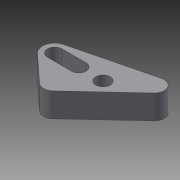
# Autodesk Inventor part: brake
Saved by Autodesk Inventor 2018 (Build 220112000, 112)
## iProperties
Created: 2019-02-20
Part Number: brake
Material: 一般
Document SubType Name: Modeling
Designer: ku_sk
Density: 1 g/cm^3
Appearance: 既定
Author: ku_sk
Autodesk Inventor part; units mm, degrees
ref_plane "YZ Plane" through (0, 0, 0) normal (1, 0, 0) x (0, 1, 0)
ref_plane "XZ Plane" through (0, 0, 0) normal (0, 1, 0) x (-1, 0, 0)
ref_plane "XY Plane" through (0, 0, 0) normal (0, 0, 1) x (1, 0, 0)
sketch "スケッチ1" plane through (0, 0, 0) normal (0, 0, 1) x (1, 0, 0)
  arc A0 (-1.1412, 2.2506) -> (-0.4102, -2.4899) centre (0, 0) ccw
  line L0 (-1.1412, 2.2506) -> (18.2751, 12.0956)
  line L1 (20.825, 9.175) -> (12.1396, -3.396)
  line L2 (10.169, -4.2326) -> (-0.4102, -2.4899)
  arc A1 (20.825, 9.175) -> (18.2751, 12.0956) centre (19.1795, 10.3118) ccw
  arc A2 (10.169, -4.2326) -> (12.1396, -3.396) centre (10.4941, -2.2592) ccw
  dimension "d0" = 2
  constraints: 6 end point, 6 point on circle, 6 tangent, 3 centre point, 1 coincident, 1 equal radius
  measures "d0" radius of A1
extrude "押し出し1" add sketch "スケッチ1" along normal blind 6.5
sketch "スケッチ3" plane through (0, 0, 6.5) normal (0, 0, 1) x (1, 0, 0)
  line L0 (0, 0) -> (1, 0) construction
  line L1 (0, 1.5) -> (1, 1.5)
  line L2 (1, -1.5) -> (0, -1.5)
  arc A0 (0, 1.5) -> (0, -1.5) centre (0, 0) ccw
  arc A1 (1, -1.5) -> (1, 1.5) centre (1, 0) ccw
  point P0 (0.5, 0)
  dimension "d7" = 3
  dimension "d8" = 1
  constraints: 8 end point, 4 point on circle, 4 tangent, 2 centre point, 1 horizontal, 1 midpoint, 1 parallel
  measures "d7" distance between parallel lines of L1 L2
  measures "d8" distance of L0.start L0.end
extrude "押し出し3" cut sketch "スケッチ3" against normal blind 5
sketch "スケッチ5" plane through (0, 0, 6.5) normal (0, 0, 1) x (1, 0, 0)
  circle A0 centre (10, 0) radius 1.5
  line L0 (-7.264, 0) -> (25.9201, 0) projected
  point P0 (0, 0)
  dimension "d14" = 3
  dimension "d15" = 10
  constraints: 1 centre point, 1 point on line
  measures "d14" diameter of A0
  measures "d15" distance of point (0, 0) A0.centre
extrude "押し出し5" cut sketch "スケッチ5" against normal blind 5
